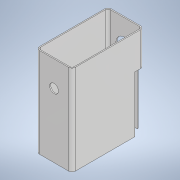
# Autodesk Inventor part: SP21V1 Tubo 40x80x100mm
Saved by Autodesk Inventor 2021.2 (Build 252289000, 289)
## iProperties
Created: 2026-06-02
Part Number: SP21V1 Tubo 40x80x100mm
Material: Aluminum
Document SubType Name: Modeling
Designer: nelso
Density: 2.7 g/cm^3
Appearance: Satin
Author: nelso
Autodesk Inventor part; units mm, degrees
ref_plane "YZ Plane" through (0, 0, 0) normal (1, 0, 0) x (0, 1, 0)
ref_plane "XZ Plane" through (0, 0, 0) normal (0, 1, 0) x (-1, 0, 0)
ref_plane "XY Plane" through (0, 0, 0) normal (0, 0, 1) x (1, 0, 0)
sketch "Sketch1" plane through (0, 0, 0) normal (0, 1, 0) x (-1, 0, 0)
  line L0 (-20, 40) -> (20, 40)
  line L1 (20, 40) -> (20, -40)
  line L2 (20, -40) -> (-20, -40)
  line L3 (-20, -40) -> (-20, 40)
  line L4 (-20, 40) -> (20, -40) construction
  line L5 (20, 40) -> (-20, -40) construction
  line L6 (-18.75, 38.75) -> (18.75, 38.75)
  line L7 (18.75, 38.75) -> (18.75, -38.75)
  line L8 (18.75, -38.75) -> (-18.75, -38.75)
  line L9 (-18.75, -38.75) -> (-18.75, 38.75)
  line L10 (-18.75, 38.75) -> (18.75, -38.75) construction
  line L11 (18.75, 38.75) -> (-18.75, -38.75) construction
  point P0 (0, 0)
  dimension "d0" = 40
  dimension "d1" = 80
  dimension "d2" = 37.5
  dimension "d3" = 77.5
  constraints: 24 end point, 4 midpoint, 4 parallel, 2 horizontal, 2 perpendicular
  measures "d0" distance of L1.end L2.end
  measures "d1" distance of L0.end L1.end
  measures "d2" distance of L7.end L8.end
  measures "d3" distance of L6.end L7.end
extrude "Extrusion1" add sketch "Sketch1" along normal mid plane 100
fillet "Fillet1" radius 3.75 4 edges at (20, 0, 40) (-20, 0, 40) (20, 0, -40) (-20, 0, -40)
fillet "Fillet1" radius 2.5 4 edges at (18.75, 0, 38.75) (-18.75, 0, -38.75) (18.75, 0, -38.75) (-18.75, 0, 38.75)
sketch "Sketch3" plane through (16.25, 50, -40) normal (0, 0, -1) x (-1, 0, 0)
  line L0 (0, 0) -> (32.5, 0) projected
  line L1 (16.25, 0) -> (16.25, -28.5)
  circle A0 centre (16.25, -28.5) radius 4.95
  point P0 (16.25, -50)
  dimension "d12" = 28.5
  dimension "d13" = 9.9
  constraints: 2 end point, 1 centre point, 1 coincident, 1 midpoint, 1 vertical
  measures "d12" distance of L1.start L1.end
  measures "d13" diameter of A0
extrude "Extrusion3" cut sketch "Sketch3" against normal through all
sketch "Sketch4" plane through (16.25, 50, -40) normal (0, 0, -1) x (-1, 0, 0)
  circle A0 centre (16.25, -28.5) radius 4.95 projected
  circle A1 centre (16.25, -28.5) radius 10
  point P0 (16.25, -50)
  dimension "d16" = 20
  constraints: 1 centre point, 1 coincident
  measures "d16" diameter of A1
extrude "Extrusion4" cut sketch "Sketch4" against normal blind 10
sketch "Sketch12" plane through (16.25, 50, -40) normal (0, 0, -1) x (-1, 0, 0)
  circle A0 centre (10.0721, -50.016) radius 3.3 projected
  circle A1 centre (10.0721, -64.016) radius 3.3 projected
  line L0 (2.55, -37.5) -> (2.55, -107.5) projected
  line L1 (2.55, -107.5) -> (-2.734, -107.5) projected
  line L2 (-2.734, -37.5) -> (2.55, -37.5) projected
  line L3 (2.55, -107.5) -> (-7.45, -107.5)
  line L4 (-7.45, -107.5) -> (-7.45, -37.5)
  line L5 (-7.45, -37.5) -> (2.55, -37.5)
  line L6 (2.55, -37.5) -> (2.55, -107.5)
  dimension "d42" = 10
  dimension "d43" = 70
  constraints: 8 end point, 2 parallel, 1 horizontal, 1 perpendicular
  measures "d42" distance of L4.end L5.end
  measures "d43" distance of L3.end L4.end
extrude "Extrusion12" cut sketch "Sketch12" against normal blind 10
body "Solid1"
